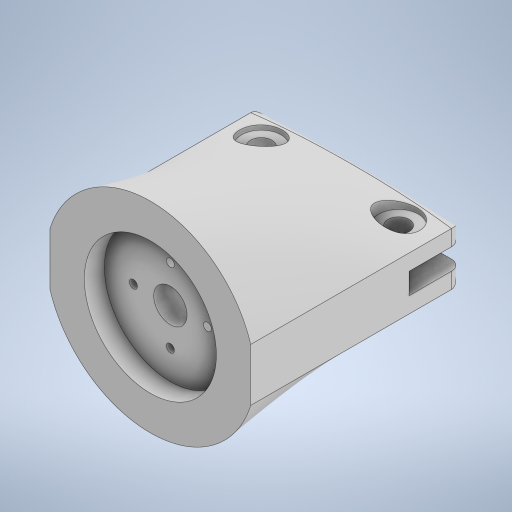
# Autodesk Inventor part: head_2
Saved by Autodesk Inventor 2023 (Build 270158000, 158)
## iProperties
Created: 2024-07-21
Part Number: head_2
Material: Generic
Document SubType Name: Modeling
Designer: Swoby
Density: 1 g/cm^3
Appearance: Default
Author: Swoby
Autodesk Inventor part; units mm, degrees
ref_plane "YZ Plane" through (0, 0, 0) normal (1, 0, 0) x (0, 1, 0)
ref_plane "XZ Plane" through (0, 0, 0) normal (0, 1, 0) x (-1, 0, 0)
sketch "Sketch1" plane through (0, 0, 0) normal (0, 0, 1) x (1, 0, 0)
  line L0 (-19, -5) -> (19, -5)
  line L1 (19, -5) -> (19, 5)
  line L2 (19, 5) -> (-19, 5)
  line L3 (-19, 5) -> (-19, -5)
  line L4 (-19, -5) -> (19, 5) construction
  line L5 (19, -5) -> (-19, 5) construction
  point P0 (0, 0)
  dimension "d0" = 38
  dimension "d1" = 10
  constraints: 12 end point, 2 midpoint, 2 parallel, 1 horizontal, 1 perpendicular
  measures "d0" distance of L2.end L1.end
  measures "d1" distance of L1.end L0.end
ref_plane "Work Plane1" through (0, 0, 40) normal (0, 0, 1) x (1, 0, 0)
sketch "Sketch2" plane through (0, 0, 40) normal (0, 0, 1) x (1, 0, 0)
  line L0 (-19, 5) -> (-19, -5) projected
  line L1 (19, 5) -> (-19, 5) construction
  line L2 (19, -5) -> (19, 5) projected
  line L3 (-19, -5) -> (19, -5) construction
  arc A0 (19, 5) -> (-19, 5) centre (0, -0.8929) ccw
  arc A1 (-19, -5) -> (19, -5) centre (0, 0.8929) ccw
  point P0 (0, 0)
  point P1 (0, -19)
  point P2 (0, 19)
  dimension "d6" = 38
  dimension "d7" = 19
  constraints: 6 point on circle, 2 centre point
  measures "d6" distance of point (0, -19) point (0, 19)
  measures "d7" distance of point (0, 19) point (0, 0)
loft "Loft1" add profiles "Sketch1", "Sketch2"
fillet "Fillet1" radius 2 4 edges at (0, 5, 0) (-19, 0, 0) (0, -5, 0) (19, 0, 0)
sketch "Sketch3" plane through (19, -5, 40) normal (1, 0, 0) x (0, 0, -1)
  line L0 (30, 7) -> (40, 7)
  line L1 (40, 7) -> (40, 3)
  line L2 (40, 3) -> (30, 3)
  line L3 (30, 3) -> (30, 7)
  point P0 (40, 5)
  point P1 (40, 5)
  dimension "d13" = 4
  dimension "d14" = 10
  constraints: 8 end point, 2 parallel, 1 coincident, 1 horizontal, 1 midpoint, 1 perpendicular
  measures "d13" distance of L2.end L0.start
  measures "d14" distance of L0.start L0.end
extrude "Extrusion1" cut sketch "Sketch3" against normal through all
sketch "Sketch4" plane through (19, -2, 10) normal (0, 1, 0) x (1, 0, 0)
  circle A0 centre (-32, 4) radius 2
  circle A1 centre (-6, 4) radius 2
  line L0 (-38, 8) -> (-38, -30) projected
  line L1 (0, 8) -> (0, -30) projected
  line L2 (-36, 10) -> (-2, 10) projected
  point P0 (-19, 10)
  dimension "d17" = 4
  dimension "d18" = 4
  dimension "d19" = 6
  dimension "d20" = 6
  dimension "d21" = 6
  dimension "d22" = 6
  constraints: 2 centre point
  measures "d17" diameter of A0
  measures "d18" diameter of A1
  measures "d19" distance from line of L0 A0.centre
  measures "d20" distance from line of L1 A1.centre
  measures "d21" distance from line of L2 A1.centre
  measures "d22" distance from line of L2 A0.centre
extrude "Extrusion2" cut sketch "Sketch4" along normal through all both and the other way through all
ref_plane "Work Plane2" through (19, 4.5, 2) normal (0, -1, 0) x (1, 0, 0)
sketch "Sketch5" plane through (19, 4.5, 2) normal (0, -1, 0) x (1, 0, 0)
  spline S0 degree 2 poles (-4, 4) (-4, 7.4641) (-7, 5.7321) (-10, 4) (-7, 2.2679) (-4, 0.5359) (-4, 4) knots 0 0 0 0.333333 0.333333 0.666667 0.666667 1 1 1 weights 1 0.5 1 0.5 1 0.5 1 projected
  spline S1 degree 2 poles (-30, 4) (-30, 7.4641) (-33, 5.7321) (-36, 4) (-33, 2.2679) (-30, 0.5359) (-30, 4) knots 0 0 0 0.333333 0.333333 0.666667 0.666667 1 1 1 weights 1 0.5 1 0.5 1 0.5 1 projected
  circle A0 centre (-6, 4) radius 3.75
  circle A1 centre (-32, 4) radius 3.75
  circle A2 centre (-6, 4) radius 2 projected
  circle A3 centre (-32, 4) radius 2 projected
  point P0 (-19, -2)
  dimension "d26" = 7.5
  dimension "d27" = 7.5
  constraints: 2 centre point, 6 other
  measures "d26" diameter of A0
  measures "d27" diameter of A1
extrude "Extrusion3" cut sketch "Sketch5" against normal through all
ref_plane "Work Plane3" through (19, -4.5, 10) normal (0, 1, 0) x (1, 0, 0)
sketch "Sketch6" plane through (19, -4.5, 10) normal (0, 1, 0) x (1, 0, 0)
  spline S0 degree 2 poles (-4, 4) (-4, 7.4641) (-7, 5.7321) (-10, 4) (-7, 2.2679) (-4, 0.5359) (-4, 4) knots 0 0 0 0.333333 0.333333 0.666667 0.666667 1 1 1 weights 1 0.5 1 0.5 1 0.5 1 projected
  line L0 (-4.0659, 7.35) -> (-2.1318, 4)
  line L1 (-2.1318, 4) -> (-4.0659, 0.65)
  line L2 (-4.0659, 0.65) -> (-7.9341, 0.65)
  line L3 (-7.9341, 0.65) -> (-9.8682, 4)
  line L4 (-9.8682, 4) -> (-7.9341, 7.35)
  line L5 (-7.9341, 7.35) -> (-4.0659, 7.35)
  line L6 (-33.9341, 7.35) -> (-30.0659, 7.35)
  line L7 (-30.0659, 7.35) -> (-28.1318, 4)
  line L8 (-28.1318, 4) -> (-30.0659, 0.65)
  line L9 (-30.0659, 0.65) -> (-33.9341, 0.65)
  line L10 (-33.9341, 0.65) -> (-35.8682, 4)
  line L11 (-35.8682, 4) -> (-33.9341, 7.35)
  circle A0 centre (-6, 4) radius 2 projected
  circle A1 centre (-32, 4) radius 2 projected
  point P0 (-19, 10)
  dimension "d31" = 6.7
  dimension "d32" = 6.7
  constraints: 24 end point, 2 coincident, 2 horizontal, 30 other
  measures "d31" distance between parallel lines of L9 L6
  measures "d32" distance between parallel lines of L2 L5
extrude "Extrusion4" cut sketch "Sketch6" against normal through all contours L0 L1 L2 L3 L4 L5 | L6 L7 L8 L9 L10 L11 | A1
sketch "Sketch8" plane through (0, 0.8929, 40) normal (0, 0, 1) x (1, 0, 0)
  circle A0 centre (0, -0.8929) radius 12.5
  dimension "d35" = 25
  constraints: 1 centre point, 1 coincident
  measures "d35" diameter of A0
extrude "Extrusion5" cut sketch "Sketch8" against normal blind 3.8
sketch "Sketch9" plane through (0, 0, 36.2) normal (0, 0, 1) x (1, 0, 0)
  line L0 (-7, 0) -> (7, 0) construction
  circle A0 centre (0, 0) radius 12.5 projected
  circle A1 centre (0, 0) radius 12.5 projected
  line L1 (0, -7) -> (0, 7) construction
  circle A2 centre (0, 7) radius 0.75
  circle A3 centre (-7, 0) radius 0.75
  circle A4 centre (7, 0) radius 0.75
  circle A5 centre (0, -7) radius 0.75
  dimension "d48" = 14
  dimension "d49" = 14
  dimension "d50" = 1.5
  dimension "d52" = 1.5
  dimension "d53" = 1.5
  dimension "d54" = 1.5
  constraints: 5 coincident, 4 centre point, 4 end point, 2 midpoint, 1 horizontal, 1 vertical
  measures "d48" distance of L0.start L0.end
  measures "d49" distance of L1.start L1.end
  measures "d50" diameter of A2
  measures "d52" diameter of A3
  measures "d53" diameter of A4
  measures "d54" diameter of A5
extrude "Extrusion6" cut sketch "Sketch9" against normal blind 7 contours A2 | A3 | A4 | A5
sketch "Sketch10" plane through (0, 0, 36.2) normal (0, 0, 1) x (1, 0, 0)
  circle A0 centre (0, 0) radius 3.15
  dimension "d55" = 6.3
  constraints: 1 centre point, 1 coincident
  measures "d55" diameter of A0
extrude "Extrusion7" cut sketch "Sketch10" against normal through all
equation "\"d7\" = 0.5 * d6"
equation "\"d17\" = d18"
equation "\"d27\" = d26"
equation "\"d32\" = d31"
body "Solid1"
